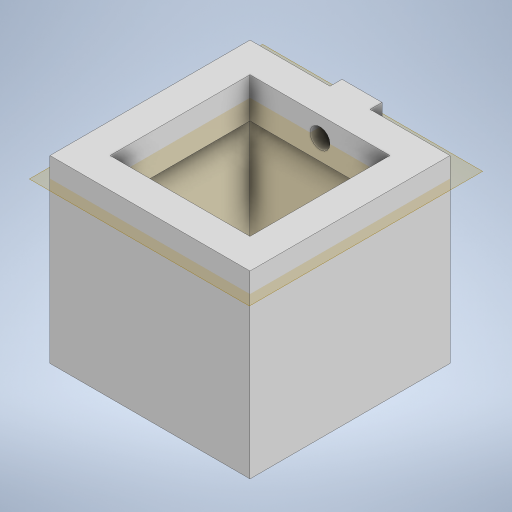
# Autodesk Inventor part: Pudelko
Saved by Autodesk Inventor 2024 (Build 280153000, 153)
## iProperties
Created: 2023-10-17
Part Number: Pudelko
Material: Generic
Document SubType Name: Modeling
Designer: Piter
Density: 1 g/cm^3
Appearance: Default
Author: Piter
Autodesk Inventor part; units mm, degrees
ref_plane "YZ Plane" through (0, 0, 0) normal (1, 0, 0) x (0, 1, 0)
ref_plane "XZ Plane" through (0, 0, 0) normal (0, 1, 0) x (-1, 0, 0)
ref_plane "XY Plane" through (0, 0, 0) normal (0, 0, 1) x (1, 0, 0)
sketch "Sketch1" plane through (0, 0, 0) normal (0, 1, 0) x (-1, 0, 0)
  line L0 (-25, -25) -> (25, -25)
  line L1 (25, -25) -> (25, 25)
  line L2 (25, 25) -> (-25, 25)
  line L3 (-25, 25) -> (-25, -25)
  line L4 (-25, -25) -> (25, 25) construction
  line L5 (25, -25) -> (-25, 25) construction
  line L6 (-22.5, 22.5) -> (22.5, 22.5)
  line L7 (22.5, 22.5) -> (22.5, -22.5)
  line L8 (22.5, -22.5) -> (-22.5, -22.5)
  line L9 (-22.5, -22.5) -> (-22.5, 22.5)
  line L10 (-22.5, 22.5) -> (22.5, -22.5) construction
  line L11 (22.5, 22.5) -> (-22.5, -22.5) construction
  point P0 (0, 0)
  dimension "d0" = 50
  dimension "d1" = 50
  dimension "d2" = 45
  dimension "d3" = 45
  constraints: 24 end point, 4 midpoint, 4 parallel, 2 horizontal, 2 perpendicular
  measures "d0" distance of L2.end L1.end
  measures "d1" distance of L1.end L0.end
  measures "d2" distance of L7.end L8.end
  measures "d3" distance of L6.end L7.end
extrude "Extrusion1" add sketch "Sketch1" along normal blind 5 contours L6 L7 L8 L9
extrude "Extrusion2" add sketch "Sketch1" along normal blind 45
sketch "Sketch2" plane through (0, 45, 0) normal (0, 1, 0) x (1, 0, 0)
  line L0 (22.5, 22.5) -> (22.5, -22.5) projected
  line L1 (-22.5, -22.5) -> (22.5, -22.5)
  line L2 (22.5, -22.5) -> (22.5, 22.5)
  line L3 (22.5, 22.5) -> (-22.5, 22.5)
  line L4 (-22.5, 22.5) -> (-22.5, -22.5)
  line L5 (17.5, -17.5) -> (-17.5, -17.5)
  line L6 (-17.5, -17.5) -> (-17.5, 17.5)
  line L7 (-17.5, 17.5) -> (17.5, 17.5)
  line L8 (17.5, 17.5) -> (17.5, -17.5)
  line L9 (17.5, -17.5) -> (-17.5, 17.5) construction
  line L10 (-17.5, -17.5) -> (17.5, 17.5) construction
  point P0 (0, 0)
  dimension "d8" = 35
  dimension "d9" = 35
  constraints: 20 end point, 4 parallel, 2 horizontal, 2 midpoint, 2 perpendicular
  measures "d8" distance of L6.end L7.end
  measures "d9" distance of L5.end L6.end
extrude "Extrusion3" add sketch "Sketch2" against normal blind 10
sketch "Sketch3" plane through (25, 0, -25) normal (0, 0, -1) x (-1, 0, 0)
  line L0 (50, 45) -> (0, 45) projected
  line L1 (25, 45) -> (25, 0)
  line L2 (20, 0) -> (30, 0)
  line L3 (30, 0) -> (30, 45)
  line L4 (30, 45) -> (20, 45)
  line L5 (20, 45) -> (20, 0)
  line L6 (20, 0) -> (30, 45) construction
  line L7 (30, 0) -> (20, 45) construction
  point P0 (25, 22.5)
  dimension "d12" = 10
  constraints: 14 end point, 4 midpoint, 2 parallel, 1 horizontal, 1 perpendicular, 1 point on line, 1 vertical
  measures "d12" distance of L4.end L3.end
extrude "Extrusion4" add sketch "Sketch3" along normal blind 3
sketch "Sketch4" plane through (-17.5, 45, -17.5) normal (0, 0, 1) x (1, 0, 0)
  line L0 (0, 0) -> (35, 0) projected
  line L1 (17.5, 0) -> (17.5, -10)
  line L2 (35, -10) -> (0, -10) projected
  circle A0 centre (17.5, -5) radius 2.5
  point P0 (17.5, -45)
  dimension "d15" = 5
  constraints: 3 midpoint, 2 end point, 1 centre point
  measures "d15" diameter of A0
extrude "Extrusion5" cut sketch "Sketch4" against normal blind 10
ref_plane "Work Plane1" through (0, 40, 0) normal (0, 1, 0) x (1, 0, 0)
body "Solid1"
